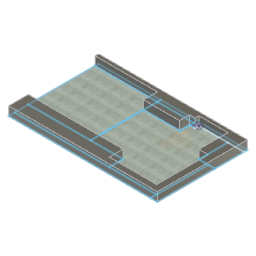
_Room Dimensions v1.5730109b-0f74-44d3-ae69-74941c8c4ce9 (Autodesk Fusion 360 design; units mm, degrees)
Autodesk Fusion 360 part; units mm, degrees
sketch "Sketch1" plane through (0, 0, 0) normal (0, 0, 1) x (1, 0, 0)
  line L0 (0, 0) -> (2133.6, 0)
  line L1 (2133.6, 0) -> (2133.6, -2133.6)
  line L2 (2133.6, -2133.6) -> (2819.4, -2133.6)
  line L3 (2819.4, -2133.6) -> (2819.4, -5918.2)
  line L4 (2819.4, -5918.2) -> (-660.4, -5918.2)
  line L5 (-660.4, -5918.2) -> (-660.4, -4902.2)
  line L6 (0, 0) -> (0, -279.4)
  line L7 (0, -279.4) -> (-406.4, -279.4)
  line L8 (-660.4, -4902.2) -> (-3048, -4902.2)
  line L9 (-3048, -4902.2) -> (-3048, -3670.2305)
  line L10 (-406.4, -1016) -> (-3048, -1016)
  line L11 (-3048, -1016) -> (-3048, -3670.2305)
  line L12 (-406.4, -279.4) -> (-406.4, -1016)
  line L13 (-3048, -1016) -> (-381, -1016)
  line L14 (-381, -1016) -> (-381, 0)
  line L15 (-381, 0) -> (-3048, 0)
  line L16 (-3048, 0) -> (-3048, -1016)
  line L17 (-381, 0) -> (0, 0)
  line L18 (0, 0) -> (0, -279.4)
  line L19 (0, -279.4) -> (-381, -279.4)
  line L20 (-381, -279.4) -> (-381, 0)
  line L21 (-3048, 0) -> (3302, 0)
  line L22 (3302, 0) -> (3302, 254)
  line L23 (3302, 254) -> (-3048, 254)
  line L24 (-3048, 254) -> (-3048, 0)
  line L25 (2133.6, 0) -> (3302, 0)
  line L26 (3302, 0) -> (3302, -2133.6)
  line L27 (3302, -2133.6) -> (2133.6, -2133.6)
  line L28 (2133.6, -2133.6) -> (2133.6, 0)
  line L29 (2819.4, -2133.6) -> (3302, -2133.6)
  line L30 (3302, -2133.6) -> (3302, -6349.9999)
  line L31 (3302, -6349.9999) -> (2819.4, -6349.9999)
  line L32 (2819.4, -6349.9999) -> (2819.4, -2133.6)
  line L33 (2819.4, -6349.9999) -> (-7616.4691, -6349.9999)
  line L34 (-7616.4691, -6349.9999) -> (-7616.4691, -5918.2)
  line L35 (-7616.4691, -5918.2) -> (2819.4, -5918.2)
  line L36 (2819.4, -5918.2) -> (2819.4, -6349.9999)
  line L37 (-660.4, -5918.2) -> (-7616.4691, -5918.2)
  line L38 (-7616.4691, -5918.2) -> (-7616.4691, -4908.0872)
  line L39 (-7616.4691, -4908.0872) -> (-660.4, -4908.0872)
  line L40 (-660.4, -4908.0872) -> (-660.4, -5918.2)
  line L41 (-3048, 254) -> (-7619.9999, 254)
  line L42 (-7619.9999, 254) -> (-7619.9999, 0)
  line L43 (-7619.9999, 0) -> (-3048, 0)
  line L44 (-3048, 0) -> (-3048, 254)
  line L45 (-7619.9999, 0) -> (-3048, 0)
  line L46 (-3048, 0) -> (-3048, -4902.2)
  line L47 (-3048, -4902.2) -> (-7619.9999, -4902.2)
  line L48 (-7619.9999, -4902.2) -> (-7619.9999, 0)
  constraint coincident L0.start L6.start
  constraint horizontal L0
  constraint perpendicular L0 L1
  constraint perpendicular L1 L2
  constraint perpendicular L2 L3
  constraint perpendicular L3 L4
  constraint perpendicular L4 L5
  constraint perpendicular L0 L6
  constraint perpendicular L6 L7
  constraint perpendicular L5 L8
  constraint perpendicular L10 L11
  constraint perpendicular L10 L12
  constraint horizontal L13
  constraint vertical L14
  constraint horizontal L15
  constraint vertical L16
  constraint horizontal L17
  constraint vertical L18
  constraint horizontal L19
  constraint vertical L20
  constraint horizontal L21
  constraint vertical L22
  constraint horizontal L23
  constraint vertical L24
  constraint horizontal L25
  constraint vertical L26
  constraint horizontal L27
  constraint vertical L28
  constraint horizontal L29
  constraint vertical L30
  constraint horizontal L31
  constraint vertical L32
  constraint horizontal L33
  constraint vertical L34
  constraint horizontal L35
  constraint vertical L36
  constraint horizontal L37
  constraint vertical L38
  constraint horizontal L39
  constraint vertical L40
  constraint horizontal L41
  constraint vertical L42
  constraint horizontal L43
  constraint vertical L44
  constraint horizontal L45
  constraint vertical L46
  constraint horizontal L47
  constraint vertical L48
extrude "Extrude1" add sketch "Sketch1" along normal blind 635 contours L0 L15 L17 L21 L22 L23 L24 L25 L44 | L1 L2 L21 L25 L26 L27 L28 L29 | L24 L41 L42 L43 L44 L45 | L3 L27 L29 L30 L31 L32 L36 | L4 L32 L33 L34 L35 L36 L37 | L5 L35 L37 L38 L39 L40
sketch "Sketch2" plane through (0, 0, 0) normal (0, 0, -1) x (1, 0, 0)
  line L0 (-7619.9999, -254) -> (3302, -254)
  line L1 (3302, -254) -> (3302, 6349.9999)
  line L2 (3302, 6349.9999) -> (-7616.4691, 6349.9999)
  line L3 (-7616.4691, 6349.9999) -> (-7616.4691, 4908.0872)
  line L4 (-7616.4691, 4908.0872) -> (-660.4, 4908.0872)
  line L5 (-660.4, 4908.0872) -> (-660.4, 5918.2)
  line L6 (-660.4, 5918.2) -> (2819.4, 5918.2)
  line L7 (2819.4, 5918.2) -> (2819.4, 2133.6)
  line L8 (2819.4, 2133.6) -> (2133.6, 2133.6)
  line L9 (2133.6, 2133.6) -> (2133.6, 0)
  line L10 (2133.6, 0) -> (-7619.9999, 0)
  line L11 (-7619.9999, 0) -> (-7619.9999, -254)
  line L12 (3302, -254) -> (-7616.4691, -254)
  line L13 (-7616.4691, -254) -> (-7616.4691, 6349.9999)
  line L14 (-7616.4691, 6349.9999) -> (3302, 6349.9999)
  line L15 (3302, 6349.9999) -> (3302, -254)
  constraint horizontal L12
  constraint vertical L13
  constraint horizontal L14
  constraint vertical L15
  constraint coincident L2.end L3.start
  constraint coincident L0.end L1.start
extrude "Extrude2" add sketch "Sketch2" along normal blind 25.4 contours L0 L1 L2 L3 L4 L5 L6 L7 L8 L9 L10 L12 L13 L14 L15 | L4 L5 L6 L7 L8 L9 L10 L13
extrude "Extrude3" add sketch "Sketch1" along normal blind 635 contours L6 L7 L14 L17 L18 L19 L20 L21 | L7 L10 L12 L13 L14 L15 L16 L20 L21 L46
sketch "Sketch3" plane through (0, 0, 0) normal (0, 0, 1) x (1, 0, 0)
  circle A0 centre (-5079.9999, 2540) radius 660.4
  circle A1 centre (-5079.9999, 2540) radius 965.2
  line L0 (-6349.9999, 2844.8) -> (-3809.9999, 2844.8)
  line L1 (-3809.9999, 2844.8) -> (-3809.9999, 2235.2)
  line L2 (-3809.9999, 2235.2) -> (-6349.9999, 2235.2)
  line L3 (-6349.9999, 2235.2) -> (-6349.9999, 2844.8)
  line L4 (-6349.9999, 2844.8) -> (-3809.9999, 2235.2) construction
  line L5 (-3809.9999, 2844.8) -> (-6349.9999, 2235.2) construction
  line L6 (-4775.1999, 3810) -> (-5384.7999, 3810)
  line L7 (-5384.7999, 3810) -> (-5384.7999, 1270)
  line L8 (-5384.7999, 1270) -> (-4775.1999, 1270)
  line L9 (-4775.1999, 1270) -> (-4775.1999, 3810)
  line L10 (-4775.1999, 3810) -> (-5384.7999, 1270) construction
  line L11 (-5384.7999, 3810) -> (-4775.1999, 1270) construction
  line L12 (-6349.9999, 2235.2) -> (-3845.6793, 2235.2)
  line L13 (-3845.6793, 2235.2) -> (-3845.6793, 2133.6)
  line L14 (-3845.6793, 2133.6) -> (-6349.9999, 2133.6)
  line L15 (-6349.9999, 2133.6) -> (-6349.9999, 2235.2)
  line L16 (-6349.9999, 2844.8) -> (-3809.9999, 2844.8)
  line L17 (-3809.9999, 2844.8) -> (-3809.9999, 2946.4)
  line L18 (-3809.9999, 2946.4) -> (-6349.9999, 2946.4)
  line L19 (-6349.9999, 2946.4) -> (-6349.9999, 2844.8)
  line L20 (-5384.7999, 3810) -> (-5486.3999, 3810)
  line L21 (-5486.3999, 3810) -> (-5486.3999, 1270)
  line L22 (-5486.3999, 1270) -> (-5384.7999, 1270)
  line L23 (-5384.7999, 1270) -> (-5384.7999, 3810)
  line L24 (-4775.1999, 1270) -> (-4673.5999, 1270)
  line L25 (-4673.5999, 1270) -> (-4673.5999, 3809.9999)
  line L26 (-4673.5999, 3809.9999) -> (-4775.1999, 3809.9999)
  line L27 (-4775.1999, 3809.9999) -> (-4775.1999, 1270)
  circle A2 centre (-5079.9999, 2540) radius 558.8
  circle A3 centre (-5079.9999, 2540) radius 1117.6
  point P0 (-5079.9999, 2540)
  point P1 (-5079.9999, 2540)
  dimension "d17" = 1320.8
  dimension "d18" = 1930.4
  dimension "d19" = 2540
  dimension "d20" = 609.6
  dimension "d21" = 609.6
  dimension "d22" = 2540
  dimension "d23" = 101.6
  dimension "d24" = 101.6
  dimension "d25" = 101.6
  dimension "d26" = 101.6
  dimension "d27" = 1117.6
  dimension "d28" = 2235.2
  constraint concentric A0 A1
  constraint horizontal L0
  constraint perpendicular L0 L1
  constraint parallel L0 L2
  constraint parallel L1 L3
  constraint coincident L4 P1
  constraint coincident L5 P1
  constraint coincident P0 A0.centre
  constraint horizontal L6
  constraint perpendicular L6 L7
  constraint parallel L6 L8
  constraint parallel L7 L9
  constraint coincident L10 P1
  constraint coincident L11 P1
  constraint coincident P1 P0
  constraint horizontal L12
  constraint vertical L13
  constraint horizontal L14
  constraint vertical L15
  constraint horizontal L16
  constraint vertical L17
  constraint horizontal L18
  constraint vertical L19
  constraint horizontal L20
  constraint vertical L21
  constraint horizontal L22
  constraint vertical L23
  constraint horizontal L24
  constraint vertical L25
  constraint horizontal L26
  constraint vertical L27
  constraint concentric A0 A2
  constraint concentric A1 A3
  measures "d17" diameter of A0
  measures "d18" diameter of A1
  measures "d19" distance of L1.end L2.end
  measures "d20" distance of L0.end L1.end
  measures "d21" distance of L7.end L8.end
  measures "d22" distance of L6.end L7.end
  measures "d23" distance of L2.end L14.end
  measures "d24" distance of L0.start L18.end
  measures "d25" distance of L6.end L20.end
  measures "d26" distance of L8.end L24.end
  measures "d27" diameter of A2
  measures "d28" diameter of A3
sketch "Sketch4" plane through (0, 0, 0) normal (0, 0, 1) x (1, 0, 0)
  circle A0 centre (-662.532, 1929.7788) radius 660.4
  circle A1 centre (-662.532, 1929.7788) radius 1270
  circle A2 centre (-662.532, 1929.7788) radius 558.8
  circle A3 centre (-662.532, 1929.7788) radius 1371.6
  line L0 (-662.532, 1929.7788) -> (-2034.132, 1929.7788)
  line L1 (-662.532, 1929.7788) -> (-1632.3996, 959.9111)
  dimension "d33" = 1320.8
  dimension "d34" = 2540
  dimension "d35" = 1117.6
  dimension "d36" = 2743.2
  dimension "d37" = 135
  constraint concentric A0 A1
  constraint concentric A0 A2
  constraint concentric A1 A3
  constraint coincident A0.centre A1.centre
  constraint coincident A3 L0.end
  constraint horizontal L0
  constraint coincident A3 L1.end
  measures "d33" diameter of A0
  measures "d34" diameter of A1
  measures "d35" diameter of A2
  measures "d36" diameter of A3
  measures "d37" angle of L0 L1
sketch "Sketch7" plane through (0, 0, 0) normal (0, 0, 1) x (1, 0, 0)
  circle A0 centre (-662.532, 1929.7788) radius 660.4
  circle A1 centre (-662.532, 1929.7788) radius 558.8
  circle A2 centre (-662.532, 1929.7788) radius 1270
  circle A3 centre (-662.532, 1929.7788) radius 1371.6
  line L0 (-662.532, 1929.7788) -> (-2034.132, 1929.7788)
  line L1 (-662.532, 1929.7788) -> (-662.532, 3301.3788)
  dimension "d42" = 1320.8
  dimension "d43" = 2540
  dimension "d44" = 1117.6
  dimension "d45" = 2743.2
  constraint concentric A0 A2
  constraint concentric A0 A1
  constraint concentric A2 A3
  constraint coincident A0.centre A1.centre
  constraint coincident L0.end A3
  constraint horizontal L0
  constraint coincident A3 L1.end
  constraint perpendicular L0 L1
  measures "d42" diameter of A0
  measures "d43" diameter of A2
  measures "d44" diameter of A1
  measures "d45" diameter of A3
component "52 dia 45" placed x (1, 0, 0) y (0, 1, 0) z (0, 0, 1) at (-651.3455, 1373.3394, 2024.6849)
component "52 dia 90" placed x (1, 0, 0) y (0, 1, 0) z (0, 0, 1) at (0, 0, 0)
